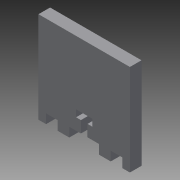
# Autodesk Inventor part: screwlockgen
Saved by Autodesk Inventor 2014 (Build 180170000, 170)
## iProperties
Created: 2014-07-13
Part Number: screwlockgen
Material: Generic
Document SubType Name: Modeling
Designer: cruiser
Density: 1 g/cm^3
Appearance: Default
Author: cruiser
Autodesk Inventor part; units mm, degrees
ref_plane "YZ Plane" through (0, 0, 0) normal (1, 0, 0) x (0, 1, 0)
ref_plane "XZ Plane" through (0, 0, 0) normal (0, 1, 0) x (-1, 0, 0)
ref_plane "XY Plane" through (0, 0, 0) normal (0, 0, 1) x (1, 0, 0)
sketch "Sketch1" plane through (0, 0, 0) normal (0, 1, 0) x (-1, 0, 0)
  line L0 (25, -25) -> (-25, -25)
  line L1 (-25, -25) -> (-25, 25)
  line L2 (-25, 25) -> (25, 25)
  line L3 (25, 25) -> (25, -25)
  line L4 (25, -25) -> (-25, 25) construction
  line L5 (-25, -25) -> (25, 25) construction
  point P0 (0, 0)
  dimension "d0" = 50
  dimension "d1" = 50
  constraints: 12 end point, 2 midpoint, 2 parallel, 1 horizontal, 1 perpendicular
  measures "d0" distance of L1.end L2.end
  measures "d1" distance of L0.end L1.end
extrude "Extrusion1" add sketch "Sketch1" along normal blind 6.35
sketch "Sketch2" plane through (0, 6.35, 0) normal (0, 1, 0) x (1, 0, 0)
  line L0 (25, 25) -> (-25, 25) projected
  line L1 (0, 0) -> (0, 25)
  line L2 (-1.8034, 25) -> (1.8034, 25)
  line L3 (1.8034, 25) -> (1.8034, 10.3)
  line L4 (1.8034, 10.3) -> (-1.8034, 10.3)
  line L5 (-1.8034, 10.3) -> (-1.8034, 25)
  line L6 (-4.4688, 13.57) -> (4.4687, 13.57)
  line L7 (4.4687, 13.57) -> (4.4687, 9.7919)
  line L8 (4.4687, 9.7919) -> (-4.4688, 9.7919)
  line L9 (-4.4688, 9.7919) -> (-4.4688, 13.57)
  line L10 (1.8034, 25) -> (8.1534, 25)
  line L11 (8.1534, 25) -> (8.1534, 19.92)
  line L12 (8.1534, 19.92) -> (1.8034, 19.92)
  line L13 (1.8034, 19.92) -> (1.8034, 25)
  line L14 (-1.8034, 25) -> (-8.1534, 25)
  line L15 (-8.1534, 25) -> (-8.1534, 19.92)
  line L16 (-8.1534, 19.92) -> (-1.8034, 19.92)
  line L17 (-1.8034, 19.92) -> (-1.8034, 25)
  line L18 (14.5034, 25) -> (20.8534, 25)
  line L19 (20.8534, 25) -> (20.8534, 19.92)
  line L20 (20.8534, 19.92) -> (14.5034, 19.92)
  line L21 (14.5034, 19.92) -> (14.5034, 25)
  line L22 (-20.8534, 25) -> (-14.5034, 25)
  line L23 (-14.5034, 25) -> (-14.5034, 19.92)
  line L24 (-14.5034, 19.92) -> (-20.8534, 19.92)
  line L25 (-20.8534, 19.92) -> (-20.8534, 25)
  dimension "d4" = 3.6068
  dimension "d5" = 3.7781
  dimension "d6" = 11.43
  dimension "d7" = 14.7
  dimension "d8" = 8.9375
  dimension "d11" = 6.35
  dimension "d12" = 5.08
  dimension "d13" = 6.35
  dimension "d14" = 5.08
  dimension "d15" = 6.35
  dimension "d16" = 5.08
  dimension "d17" = 6.35
  dimension "d18" = 6.35
  dimension "d19" = 5.08
  dimension "d20" = 6.35
  constraints: 50 end point, 12 parallel, 6 horizontal, 6 perpendicular, 3 point on line, 1 midpoint, 2 other
  measures "d4" distance between parallel lines of L3 L5
  measures "d5" distance between parallel lines of L8 L6
  measures "d6" distance between parallel lines of L0 L6
  measures "d7" distance of L4.end L2.start
  measures "d8" distance between parallel lines of L9 L7
  measures "d11" distance of L11.end L12.end
  measures "d12" distance of L10.end L11.end
  measures "d13" distance of L16.end L15.end
  measures "d14" distance of L15.end L14.end
  measures "d15" distance of L19.end L20.end
  measures "d16" distance of L18.end L19.end
  measures "d17" distance between parallel lines of L11 L21
  measures "d18" distance of L23.end L24.end
  measures "d19" distance of L22.end L23.end
  measures "d20" distance between parallel lines of L15 L23
extrude "6-32 tslot" cut sketch "Sketch2" against normal up to next
equation "\"d12\" = m2_thickness"
equation "\"d14\" = m2_thickness"
equation "\"d16\" = m2_thickness"
equation "\"d19\" = m2_thickness"
equation "\"m2_thickness\" = 5.08"
body "Solid1"
